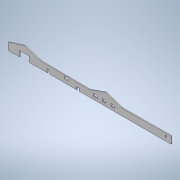
# Autodesk Inventor part: unwrappedBarnAboveCementRocks
Saved by Autodesk Inventor 2020.1 (Build 241239000, 239)
## iProperties
Created: 2019-08-11
Part Number: unwrappedBarnAboveCementRocks
Material: Generic
Document SubType Name: Modeling
Designer: steele
Density: 1 g/cm^3
Appearance: Default
Mass: 5.01434e+07 g
Surface Area: 3.77135e+06 cm^2
Volume: 5.01434e+07 cm^3
Author: steele
Autodesk Inventor part; units mm, degrees
ref_plane "YZ Plane" through (0, 0, 0) normal (1, 0, 0) x (0, 1, 0)
ref_plane "XZ Plane" through (0, 0, 0) normal (0, 1, 0) x (-1, 0, 0)
ref_plane "XY Plane" through (0, 0, 0) normal (0, 0, 1) x (1, 0, 0)
sketch "Sketch1" plane through (0, 0, 0) normal (0, 0, 1) x (1, 0, 0)
  line L0 (0, 0) -> (0, 2616.2)
  line L1 (0, 0) -> (4267.2, 0)
  line L2 (4267.2, 0) -> (4267.2, 2133.6)
  line L3 (4267.2, 2133.6) -> (7899.4, 2133.6)
  line L4 (7899.4, 2133.6) -> (7899.4, 25.4)
  line L5 (7899.4, 25.4) -> (12141.2, 25.4)
  line L6 (12141.2, 25.4) -> (12141.2, 2616.2)
  line L7 (12141.2, 2616.2) -> (0, 2616.2) construction
  line L8 (6070.6, 2616.2) -> (6070.6, 6494.6516) construction
  line L9 (0, 2616.2) -> (6070.6, 4572)
  line L10 (12141.2, 2616.2) -> (6070.6, 4572)
  line L11 (12141.2, 25.4) -> (30429.2, 25.4)
  line L12 (30429.2, 25.4) -> (30429.2, 2463.8)
  line L13 (30429.2, 2463.8) -> (12141.2, 2616.2)
  line L14 (14622.9659, 25.4) -> (15588.1659, 25.4)
  line L15 (15588.1659, 25.4) -> (15588.1659, 1469.803)
  line L16 (15588.1659, 1469.803) -> (14622.9659, 1469.803)
  line L17 (14622.9659, 1469.803) -> (14622.9659, 25.4)
  line L18 (21005.8, 2180.6143) -> (22529.8, 2180.6143)
  line L19 (22529.8, 2180.6143) -> (22529.8, 1266.2143)
  line L20 (22529.8, 1266.2143) -> (21005.8, 1266.2143)
  line L21 (21005.8, 1266.2143) -> (21005.8, 2180.6143)
  line L22 (21005.8, 2180.6143) -> (22529.8, 1266.2143) construction
  line L23 (22529.8, 2180.6143) -> (21005.8, 1266.2143) construction
  line L24 (30429.2, 25.4) -> (42621.2, 25.4)
  line L25 (42621.2, 25.4) -> (42621.2, 2565.4)
  line L26 (36525.2, 25.4) -> (36525.2, 4597.4) construction
  line L27 (30429.2, 2463.8) -> (36525.2, 4597.4)
  line L28 (42621.2, 2565.4) -> (36525.2, 4597.4)
  line L29 (31954.9483, 1152.8729) -> (33478.9483, 1152.8729)
  line L30 (33478.9483, 1152.8729) -> (33478.9483, 2041.8729)
  line L31 (33478.9483, 2041.8729) -> (31954.9483, 2041.8729)
  line L32 (31954.9483, 2041.8729) -> (31954.9483, 1152.8729)
  line L33 (31954.9483, 1152.8729) -> (33478.9483, 2041.8729) construction
  line L34 (33478.9483, 1152.8729) -> (31954.9483, 2041.8729) construction
  line L35 (35384.3088, 1152.8729) -> (36603.5088, 1152.8729)
  line L36 (36603.5088, 1152.8729) -> (36603.5088, 2041.8729)
  line L37 (36603.5088, 2041.8729) -> (35384.3088, 2041.8729)
  line L38 (35384.3088, 2041.8729) -> (35384.3088, 1152.8729)
  line L39 (35384.3088, 1152.8729) -> (36603.5088, 2041.8729) construction
  line L40 (36603.5088, 1152.8729) -> (35384.3088, 2041.8729) construction
  line L41 (38591.5468, 1152.8729) -> (39810.7468, 1152.8729)
  line L42 (39810.7468, 1152.8729) -> (39810.7468, 2041.8729)
  line L43 (39810.7468, 2041.8729) -> (38591.5468, 2041.8729)
  line L44 (38591.5468, 2041.8729) -> (38591.5468, 1152.8729)
  line L45 (38591.5468, 1152.8729) -> (39810.7468, 2041.8729) construction
  line L46 (39810.7468, 1152.8729) -> (38591.5468, 2041.8729) construction
  line L47 (42621.2, 25.4) -> (60960, 25.4)
  line L48 (60960, 25.4) -> (60960, 2641.6)
  line L49 (60960, 2641.6) -> (42621.2, 2565.4)
  line L50 (59123.1327, 1254.4729) -> (58742.1327, 1254.4729)
  line L51 (58742.1327, 1254.4729) -> (58742.1327, 1940.2729)
  line L52 (58742.1327, 1940.2729) -> (59123.1327, 1940.2729)
  line L53 (59123.1327, 1940.2729) -> (59123.1327, 1254.4729)
  line L54 (59123.1327, 1254.4729) -> (58742.1327, 1940.2729) construction
  line L55 (58742.1327, 1254.4729) -> (59123.1327, 1940.2729) construction
  line L56 (25603.2, 25.4) -> (26619.2, 25.4)
  line L57 (26619.2, 25.4) -> (26619.2, 1016)
  line L58 (26619.2, 1016) -> (25603.2, 1016)
  line L59 (25603.2, 1016) -> (25603.2, 25.4)
  point P0 (21767.8, 1723.4143)
  point P1 (32716.9483, 1597.3729)
  point P2 (35993.9088, 1597.3729)
  point P3 (39201.1468, 1597.3729)
  point P4 (58932.6327, 1597.3729)
  dimension "d0" = 2616.2
  dimension "d1" = 4267.2
  dimension "d2" = 2133.6
  dimension "d3" = 3632.2
  dimension "d4" = 4241.8
  dimension "d5" = 2590.8
  dimension "d6" = 18288
  dimension "d7" = 2438.4
  dimension "d8" = 965.2
  dimension "d9" = 914.4
  dimension "d10" = 1524
  dimension "d11" = 4572
  dimension "d12" = 12192
  dimension "d13" = 2540
  dimension "d14" = 4572
  dimension "d15" = 1524
  dimension "d16" = 889
  dimension "d17" = 1219.2
  dimension "d18" = 889
  dimension "d19" = 1219.2
  dimension "d20" = 889
  dimension "d21" = 18338.8
  dimension "d22" = 2616.2
  dimension "d23" = 381
  dimension "d24" = 685.8
  dimension "d27" = 1016
  dimension "d28" = 990.6
  dimension "d29" = 3810
  dimension "d30" = 3073.4
  dimension "d33" = 60960
  dimension "d34" = 6377.8788
  dimension "d35" = 6377.8788
  dimension "d36" = 18288
  dimension "d37" = 6458.5962
  dimension "d38" = 6425.7482
  dimension "d39" = 18338.8
  constraints: 120 end point, 15 perpendicular, 14 parallel, 12 midpoint, 11 horizontal, 4 point on line, 3 vertical
  measures "d0" distance of L0.start L0.end
  measures "d1" distance of L0.start L1.end
  measures "d2" distance of L1.end L2.end
  measures "d3" distance of L2.end L3.end
  measures "d4" distance of L4.end L5.end
  measures "d5" distance of L5.end L6.end
  measures "d6" distance of L5.end L11.end
  measures "d7" distance of L11.end L12.end
  measures "d8" distance of L16.end L15.end
  measures "d9" distance of L18.end L19.end
  measures "d10" distance between parallel lines of L19 L21
  measures "d11" distance from line of L1 L9.end
  measures "d12" distance of L11.end L24.end
  measures "d13" distance of L24.end L25.end
  measures "d14" distance of L26.start L26.end
  measures "d15" distance of L29.start L29.end
  measures "d16" distance of L30.end L29.end
  measures "d17" distance of L35.start L35.end
  measures "d18" distance between parallel lines of L37 L35
  measures "d19" distance of L41.start L41.end
  measures "d20" distance of L42.end L41.end
  measures "d21" distance of L24.end L47.end
  measures "d22" distance of L47.end L48.end
  measures "d23" distance of L50.start L50.end
  measures "d24" distance of L50.end L51.end
  measures "d27" distance of L58.end L57.end
  measures "d28" distance of L56.end L57.end
  measures "d29" distance between parallel lines of L57 L12
  measures "d30" distance between parallel lines of L19 L59
  measures "d33" distance of L47.end L0.start
  measures "d34" distance of L9.end L0.end
  measures "d35" distance of L6.end L9.end
  measures "d36" horizontal distance of L12.end L6.end
  measures "d37" distance of L28.end L12.end
  measures "d38" distance of L25.end L26.end
  measures "d39" horizontal distance of L48.end L25.end
extrude "Extrusion2" add sketch "Sketch1" against normal blind 304.8 contours L0 L9 L10 L6 L5 L4 L3 L2 L1 | L13 L12 L11 L57 L58 L59 L15 L16 L17 L6 | L27 L28 L25 L24 L12 | L25 L49 L48 L47
body "Solid2"
